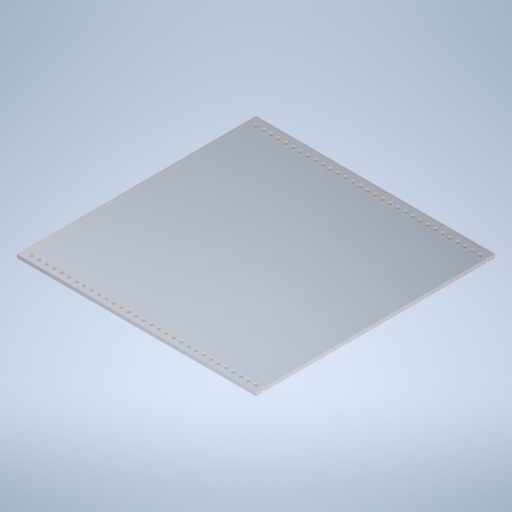
# Autodesk Inventor part: Polycarbonate-Note-Rest
Saved by Autodesk Inventor 2024 (Build 280153000, 153)
## iProperties
Created: 2024-01-23
Part Number: Polycarbonate-Note-Rest
Material: Polycarbonate, Smoke
Document SubType Name: Modeling
Designer: rohan
Density: 1.2 g/cm^3
Appearance: Polycarbonate - Smoked
Author: rohan
Autodesk Inventor part; units mm, degrees
ref_plane "YZ Plane" through (0, 0, 0) normal (1, 0, 0) x (0, 1, 0)
ref_plane "XZ Plane" through (0, 0, 0) normal (0, 1, 0) x (-1, 0, 0)
ref_plane "XY Plane" through (0, 0, 0) normal (0, 0, 1) x (1, 0, 0)
sketch "Sketch1" plane through (0, 0, 0) normal (0, 1, 0) x (-1, 0, 0)
  line L0 (279.4, 203.2) -> (-279.4, 203.2)
  line L1 (-279.4, 203.2) -> (-279.4, -203.2)
  line L2 (-279.4, -203.2) -> (279.4, -203.2)
  line L3 (279.4, -203.2) -> (279.4, 203.2)
  line L4 (279.4, 203.2) -> (-279.4, -203.2) construction
  line L5 (-279.4, 203.2) -> (279.4, -203.2) construction
  point P0 (0, 0)
  dimension "d0" = 558.8
  dimension "d1" = 406.4
  constraints: 12 end point, 2 midpoint, 2 parallel, 1 horizontal, 1 perpendicular
  measures "d0" distance of L2.end L1.end
  measures "d1" distance of L1.end L0.end
extrude "Extrusion1" add sketch "Sketch1" along normal blind 6.35
sketch "Sketch2" plane through (0, 6.35, 0) normal (0, 1, 0) x (1, 0, 0)
  circle A0 centre (-266.7, -190.5) radius 2.4892
  line L0 (-279.4, 203.2) -> (-279.4, -203.2) projected
  line L1 (-279.4, -203.2) -> (279.4, -203.2) projected
  circle A1 centre (-254, -190.5) radius 2.4892
  circle A2 centre (-241.3, -190.5) radius 2.4892
  circle A3 centre (-228.6, -190.5) radius 2.4892
  circle A4 centre (-215.9, -190.5) radius 2.4892
  circle A5 centre (-203.2, -190.5) radius 2.4892
  circle A6 centre (-190.5, -190.5) radius 2.4892
  circle A7 centre (-177.8, -190.5) radius 2.4892
  circle A8 centre (-165.1, -190.5) radius 2.4892
  circle A9 centre (-152.4, -190.5) radius 2.4892
  circle A10 centre (-139.7, -190.5) radius 2.4892
  circle A11 centre (-127, -190.5) radius 2.4892
  circle A12 centre (-114.3, -190.5) radius 2.4892
  circle A13 centre (-101.6, -190.5) radius 2.4892
  circle A14 centre (-88.9, -190.5) radius 2.4892
  circle A15 centre (-76.2, -190.5) radius 2.4892
  circle A16 centre (-63.5, -190.5) radius 2.4892
  circle A17 centre (-50.8, -190.5) radius 2.4892
  circle A18 centre (-38.1, -190.5) radius 2.4892
  circle A19 centre (-25.4, -190.5) radius 2.4892
  circle A20 centre (-12.7, -190.5) radius 2.4892
  circle A21 centre (0, -190.5) radius 2.4892
  circle A22 centre (12.7, -190.5) radius 2.4892
  circle A23 centre (25.4, -190.5) radius 2.4892
  circle A24 centre (38.1, -190.5) radius 2.4892
  circle A25 centre (50.8, -190.5) radius 2.4892
  circle A26 centre (63.5, -190.5) radius 2.4892
  circle A27 centre (76.2, -190.5) radius 2.4892
  circle A28 centre (88.9, -190.5) radius 2.4892
  circle A29 centre (101.6, -190.5) radius 2.4892
  circle A30 centre (114.3, -190.5) radius 2.4892
  circle A31 centre (127, -190.5) radius 2.4892
  circle A32 centre (139.7, -190.5) radius 2.4892
  circle A33 centre (152.4, -190.5) radius 2.4892
  circle A34 centre (165.1, -190.5) radius 2.4892
  circle A35 centre (177.8, -190.5) radius 2.4892
  circle A36 centre (190.5, -190.5) radius 2.4892
  circle A37 centre (203.2, -190.5) radius 2.4892
  circle A38 centre (215.9, -190.5) radius 2.4892
  circle A39 centre (228.6, -190.5) radius 2.4892
  circle A40 centre (241.3, -190.5) radius 2.4892
  circle A41 centre (254, -190.5) radius 2.4892
  circle A42 centre (266.7, -190.5) radius 2.4892
  line L2 (-329.0409, 0) -> (315.6584, 0) construction
  circle A43 centre (-266.7, 190.5) radius 2.4892
  circle A44 centre (-254, 190.5) radius 2.4892
  circle A45 centre (-241.3, 190.5) radius 2.4892
  circle A46 centre (-228.6, 190.5) radius 2.4892
  circle A47 centre (-215.9, 190.5) radius 2.4892
  circle A48 centre (-203.2, 190.5) radius 2.4892
  circle A49 centre (-190.5, 190.5) radius 2.4892
  circle A50 centre (-177.8, 190.5) radius 2.4892
  circle A51 centre (-165.1, 190.5) radius 2.4892
  circle A52 centre (-152.4, 190.5) radius 2.4892
  circle A53 centre (-139.7, 190.5) radius 2.4892
  circle A54 centre (-127, 190.5) radius 2.4892
  circle A55 centre (-114.3, 190.5) radius 2.4892
  circle A56 centre (-101.6, 190.5) radius 2.4892
  circle A57 centre (-88.9, 190.5) radius 2.4892
  circle A58 centre (-76.2, 190.5) radius 2.4892
  circle A59 centre (-63.5, 190.5) radius 2.4892
  circle A60 centre (-50.8, 190.5) radius 2.4892
  circle A61 centre (-38.1, 190.5) radius 2.4892
  circle A62 centre (-25.4, 190.5) radius 2.4892
  circle A63 centre (-12.7, 190.5) radius 2.4892
  circle A64 centre (0, 190.5) radius 2.4892
  circle A65 centre (12.7, 190.5) radius 2.4892
  circle A66 centre (25.4, 190.5) radius 2.4892
  circle A67 centre (38.1, 190.5) radius 2.4892
  circle A68 centre (50.8, 190.5) radius 2.4892
  circle A69 centre (63.5, 190.5) radius 2.4892
  circle A70 centre (76.2, 190.5) radius 2.4892
  circle A71 centre (88.9, 190.5) radius 2.4892
  circle A72 centre (101.6, 190.5) radius 2.4892
  circle A73 centre (114.3, 190.5) radius 2.4892
  circle A74 centre (127, 190.5) radius 2.4892
  circle A75 centre (139.7, 190.5) radius 2.4892
  circle A76 centre (152.4, 190.5) radius 2.4892
  circle A77 centre (165.1, 190.5) radius 2.4892
  circle A78 centre (177.8, 190.5) radius 2.4892
  circle A79 centre (190.5, 190.5) radius 2.4892
  circle A80 centre (203.2, 190.5) radius 2.4892
  circle A81 centre (215.9, 190.5) radius 2.4892
  circle A82 centre (228.6, 190.5) radius 2.4892
  circle A83 centre (241.3, 190.5) radius 2.4892
  circle A84 centre (254, 190.5) radius 2.4892
  circle A85 centre (266.7, 190.5) radius 2.4892
  point P0 (0, 0)
  dimension "d4" = 4.9784
  dimension "d5" = 12.7
  dimension "d6" = 12.7
  dimension "d9" = 12.7
  constraints: 86 centre point, 43 symmetric about line, 2 end point, 2 horizontal, 127 other
  measures "d4" diameter of A0
  measures "d5" distance from line of L0 A0.centre
  measures "d6" distance from line of L1 A0.centre
  measures "d9" distance of A0.centre A1.centre
extrude "Extrusion2" cut sketch "Sketch2" against normal blind 6.35
sketch "Sketch3" plane through (279.4, 0, 203.2) normal (1, 0, 0) x (0, 0, -1)
  line L0 (0, 0) -> (406.4, 0) projected
  line L1 (406.4, 0) -> (406.4, 6.35) projected
  line L2 (0, 6.35) -> (406.4, 6.35) projected
  line L3 (0, 0) -> (0, 6.35) projected
  point P0 (203.2, 0)
extrude "Extrusion3" cut sketch "Sketch3" against normal blind 152.4
body "Solid1"
